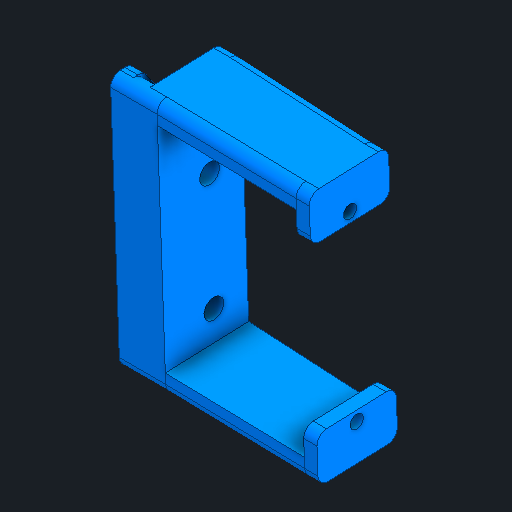
# Autodesk Inventor part: servo_mount
Saved by Autodesk Inventor 2023 (Build 270158030, 158C)
## iProperties
Created: 2022-03-29
Part Number: servo_mount
Material: Generic
Document SubType Name: Modeling
Designer: kardo
Density: 1 g/cm^3
Appearance: Blue Plastic
Author: kardo
Autodesk Inventor part; units mm, degrees
ref_plane "YZ Plane" through (0, 0, 0) normal (1, 0, 0) x (0, 1, 0)
ref_plane "XZ Plane" through (0, 0, 0) normal (0, 1, 0) x (-1, 0, 0)
ref_plane "XY Plane" through (0, 0, 0) normal (0, 0, 1) x (1, 0, 0)
derived "stencil_frame.ipt"
sketch "sk_servo_mount" plane through (-54.6, 0, 0) normal (1, 0, 0) x (0, 1, 0)
  line L0 (-241.5001, 19.2432) -> (11.22, 28.376) construction
  line L1 (-345, 3089.1136) -> (-345, -1866.0023) construction
  line L2 (0, 3089.1136) -> (0, -1866.0023) construction
  line L3 (-195.0558, 20.9216) -> (-195.2941, 27.5173) construction
  line L4 (-195.2941, 27.5173) -> (-177.3059, 28.1674) construction
  line L5 (-177.3059, 28.1674) -> (-177.0675, 21.5717) construction
  point P0 (0, 0)
  point P1 (-186.3, 27.8423)
ref_plane "plane_cowl_left" through (-54.6, 0, 0) normal (1, 0, 0) x (0, 1, 0)
derived "parameters_frame.ipt"
derived "parameters_powertrain.ipt"
derived "parameters_hardware.ipt"
ref_plane "plane_inner_stringer" through (-54.6, -241.5001, 19.2432) normal (1, 0, 0) x (0, 0.9993477, 0.0361144)
ref_plane "plane_fastening" through (-28.6, -241.5001, 19.2432) normal (1, 0, 0) x (0, 0.9993477, 0.0361144)
ref_plane "plane_servo_rod_joint" through (-14.6, -241.5001, 19.2432) normal (1, 0, 0) x (0, 0.9993477, 0.0361144)
sketch "sk_fastening" plane through (-28.6, -241.5001, 19.2432) normal (1, 0, 0) x (0, 0.9993477, 0.0361144)
  line L0 (46.4746, 6.6) -> (64.4746, 6.6) construction
  line L1 (55.4746, 6.6) -> (55.4746, 106.6) construction
  line L2 (55.4746, 106.6) -> (155.4746, 106.6) construction
  line L3 (155.4746, 106.6) -> (155.4746, 22.6) construction
  line L4 (155.4746, 22.6) -> (63.4746, 22.6) construction
  line L5 (63.4746, 22.6) -> (63.4746, 8.6) construction
  line L6 (63.4746, 8.6) -> (58.4746, 8.6) construction
  line L7 (41.9746, 14.6) -> (41.9746, 2.6)
  line L8 (41.9746, 2.6) -> (45.9746, 2.6)
  line L9 (45.9746, 2.6) -> (45.9746, 14.6)
  line L10 (45.9746, 14.6) -> (41.9746, 14.6)
  line L11 (70.9746, 14.6) -> (70.9746, 2.6)
  line L12 (70.9746, 2.6) -> (74.9746, 2.6)
  line L13 (74.9746, 2.6) -> (74.9746, 14.6)
  line L14 (74.9746, 14.6) -> (70.9746, 14.6)
  line L15 (45.9746, 14.6) -> (70.9746, 14.6) construction
  line L16 (70.9746, 2.6) -> (45.9746, 2.6) construction
  line L17 (58.4746, 2.6) -> (58.4746, 14.6) construction
  line L18 (41.9746, 14.6) -> (38.9746, 14.6)
  line L19 (38.9746, 14.6) -> (38.9746, 2.6)
  line L20 (38.9746, 2.6) -> (41.9746, 2.6)
  line L21 (74.9746, 14.6) -> (77.9746, 14.6)
  line L22 (77.9746, 14.6) -> (77.9746, 2.6)
  line L23 (77.9746, 2.6) -> (74.9746, 2.6)
  line L24 (44.4746, 8.6) -> (45.9746, 8.6) construction
  line L25 (70.9746, 8.6) -> (72.4746, 8.6) construction
  point P0 (240.6476, -27.9523)
  dimension "d46" = 100
  dimension "d47" = 84
  dimension "d49" = 100
  dimension "d50" = 92
  dimension "d52" = 14
  dimension "d53" = 5
  dimension "d54" = 25
  dimension "d55" = 33
  dimension "d56" = 3
  dimension "d57" = 3
  dimension "d58" = 12
  dimension "d59" = 28
  constraints: 50 end point, 8 collinear, 8 perpendicular, 7 parallel, 5 midpoint, 2 point on line, 1 coincident, 1 other
  measures "d46" distance of L1.end L2.end
  measures "d47" distance of L2.end L3.end
  measures "d49" distance of L1.start L1.end
  measures "d50" distance of L3.end L4.end
  measures "d52" distance of L4.end L5.end
  measures "d53" distance of L6.end L5.end
  measures "d54" distance between parallel lines of L11 L9
  measures "d55" distance between parallel lines of L13 L7
  measures "d56" distance of L7.start L18.end
  measures "d57" distance of L13.end L21.end
  measures "d58" distance of L21.end L22.end
  measures "d59" distance of L25.end L24.start
sketch "sk_base" plane through (-54.6, -241.5001, 19.2432) normal (1, 0, 0) x (0, 0.9993477, 0.0361144)
  line L0 (41.9746, 14.6) -> (38.9746, 14.6) construction
  line L1 (38.9746, 14.6) -> (38.9746, 2.6) construction
  line L2 (38.9746, 2.6) -> (41.9746, 2.6) construction
  line L3 (77.9746, 2.6) -> (74.9746, 2.6) construction
  line L4 (77.9746, 14.6) -> (77.9746, 2.6) construction
  line L5 (74.9746, 14.6) -> (77.9746, 14.6) construction
  line L6 (46.4746, 6.6) -> (64.4746, 6.6) construction
  line L7 (0, 0) -> (252.8851, 0) construction
  line L8 (38.9746, 1.5) -> (77.9746, 1.5)
  line L9 (77.9746, 1.5) -> (77.9746, 14.1)
  line L10 (77.9746, 14.1) -> (38.9746, 14.1)
  line L11 (38.9746, 14.1) -> (38.9746, 1.5)
  line L12 (46.4746, 6.6) -> (38.9746, 6.6) construction
  line L13 (46.4746, 6.6) -> (46.4746, 14.1) construction
  line L14 (64.4746, 6.6) -> (77.9746, 6.6) construction
  line L15 (64.4746, 6.6) -> (64.4746, 14.1) construction
  point P0 (240.6476, -27.9523)
  point P1 (58.4746, 8.6)
  point P2 (55.4746, 6.6)
  dimension "d60" = 22.5
  dimension "d61" = 16.5
  dimension "d62" = 18
  dimension "d64" = 1.5
  dimension "d65" = 7.5
  dimension "d66" = 16.5
  dimension "d67" = 22.5
  constraints: 16 end point, 6 perpendicular, 4 point on line, 2 parallel
  measures "d60" distance from line of L4 point (55.475, 6.6)
  measures "d61" distance from line of L1 point (55.475, 6.6)
  measures "d62" distance of L6.start L6.end
  measures "d64" distance between parallel lines of L7 L8
  measures "d65" distance of L12.start L13.end
  measures "d66" distance from line of point (55.475, 6.6) L11
  measures "d67" distance from line of point (55.475, 6.6) L9
ref_plane "plane_column_bottom" through (-52.1, -241.5001, 19.2432) normal (1, 0, 0) x (0, 0.9993477, 0.0361144)
ref_plane "plane_outer_plate" through (-57.1, -241.5001, 19.2432) normal (1, 0, 0) x (0, 0.9993477, 0.0361144)
sketch "sk_hex_holes" plane through (-57.1, -241.5001, 19.2432) normal (1, 0, 0) x (0, 0.9993477, 0.0361144)
  line L0 (48.0624, 9.35) -> (49.6501, 6.6)
  line L1 (49.6501, 6.6) -> (48.0624, 3.85)
  line L2 (48.0624, 3.85) -> (44.8869, 3.85)
  line L3 (44.8869, 3.85) -> (43.2992, 6.6)
  line L4 (43.2992, 6.6) -> (44.8869, 9.35)
  line L5 (44.8869, 9.35) -> (48.0624, 9.35)
  line L6 (66.0624, 9.35) -> (67.6501, 6.6)
  line L7 (67.6501, 6.6) -> (66.0624, 3.85)
  line L8 (66.0624, 3.85) -> (62.8869, 3.85)
  line L9 (62.8869, 3.85) -> (61.2992, 6.6)
  line L10 (61.2992, 6.6) -> (62.8869, 9.35)
  line L11 (62.8869, 9.35) -> (66.0624, 9.35)
  point P0 (240.6476, -27.9523)
  point P1 (46.4746, 6.6)
  point P2 (64.4746, 6.6)
  point P3 (46.4746, 6.6)
  point P4 (64.4746, 6.6)
  dimension "d102" = 5.5
  constraints: 24 end point, 2 coincident, 2 collinear, 26 other
  measures "d102" distance between parallel lines of L2 L5
sketch "sk_bridge" plane through (-54.6, -241.5001, 19.2432) normal (1, 0, 0) x (0, 0.9993477, 0.0361144)
  line L0 (77.9746, 14.1) -> (38.9746, 14.1) projected
  line L1 (38.9746, 14.1) -> (38.9746, 1.5) projected
  line L2 (77.9746, 1.5) -> (77.9746, 14.1) projected
  line L3 (38.9746, 11.1) -> (77.9746, 11.1)
  point P0 (240.6476, -27.9523)
  dimension "d70" = 3
  constraints: 2 end point, 2 point on line, 1 parallel
  measures "d70" distance between parallel lines of L0 L3
sketch "sk_backplate" plane through (-57.1, -241.5001, 19.2432) normal (1, 0, 0) x (0, 0.9993477, 0.0361144)
  line L0 (38.9746, 14.1) -> (38.9746, 1.5) construction
  line L1 (77.9746, 14.1) -> (38.9746, 14.1) projected
  line L2 (77.9746, 1.5) -> (77.9746, 14.1) construction
  line L3 (66.0624, 3.85) -> (62.8869, 3.85) projected
  line L4 (48.0624, 3.85) -> (44.8869, 3.85) projected
  line L5 (77.9746, 14.1) -> (77.9746, 11.1)
  line L6 (69.2378, 3.85) -> (66.0624, 3.85)
  line L7 (62.8869, 3.85) -> (48.0624, 3.85)
  line L8 (44.8869, 3.85) -> (41.7115, 3.85)
  line L9 (38.9746, 14.1) -> (38.9746, 11.1)
  line L10 (44.8869, 3.85) -> (43.2992, 6.6) construction
  line L11 (38.9746, 11.1) -> (77.9746, 11.1) construction
  line L12 (67.6501, 6.6) -> (66.0624, 3.85) construction
  line L13 (41.7115, 3.85) -> (40.1238, 6.6)
  line L14 (40.1238, 6.6) -> (38.9746, 11.1)
  line L15 (77.9746, 11.1) -> (70.8255, 6.6)
  line L16 (70.8255, 6.6) -> (69.2378, 3.85)
  point P0 (240.6476, -27.9523)
  constraints: 18 end point, 4 equal length, 2 collinear, 2 parallel
ref_plane "plane_column_top" through (-30.6, -241.5001, 19.2432) normal (1, 0, 0) x (0, 0.9993477, 0.0361144)
extrude "extrude_fastening_plates" add sketch "sk_fastening" against normal up to surface (2 mm away)
extrude "extrude_backplate" add sketch "sk_backplate" against normal blind 2
extrude "extrude_front_plate" add sketch "sk_base" along normal up to surface (2.5 mm away)
extrude "extrude_bridge" add sketch "sk_bridge" against normal up to surface (2.5 mm away)
sketch "sk_column_bottom_1" plane through (-52.1, -241.5001, 19.2432) normal (1, 0, 0) x (0, 0.9993477, 0.0361144)
  line L0 (77.9746, 14.1) -> (38.9746, 14.1) construction
  line L1 (38.9746, 1.5) -> (77.9746, 1.5) construction
  line L2 (41.9746, 14.6) -> (41.9746, 2.6) construction
  line L3 (38.9746, 14.6) -> (38.9746, 2.6) construction
  line L4 (38.9746, 14.1) -> (41.9746, 14.1)
  line L5 (41.9746, 14.1) -> (41.9746, 1.5)
  line L6 (41.9746, 1.5) -> (38.9746, 1.5)
  line L7 (38.9746, 1.5) -> (38.9746, 14.1)
  point P0 (240.6476, -27.9523)
  constraints: 8 end point, 4 collinear
sketch "sk_column_top_1" plane through (-30.6, -241.5001, 19.2432) normal (1, 0, 0) x (0, 0.9993477, 0.0361144)
  line L0 (38.9746, 14.6) -> (38.9746, 2.6) projected
  line L1 (41.9746, 14.6) -> (38.9746, 14.6) projected
  line L2 (41.9746, 14.6) -> (41.9746, 2.6) projected
  line L3 (38.9746, 2.6) -> (41.9746, 2.6) projected
  point P0 (240.6476, -27.9523)
sketch "sk_column_bottom_2" plane through (-52.1, -241.5001, 19.2432) normal (1, 0, 0) x (0, 0.9993477, 0.0361144)
  line L0 (74.9746, 2.6) -> (74.9746, 14.6) construction
  line L1 (77.9746, 14.6) -> (77.9746, 2.6) construction
  line L2 (77.9746, 14.1) -> (38.9746, 14.1) construction
  line L3 (38.9746, 1.5) -> (77.9746, 1.5) construction
  line L4 (74.9746, 14.1) -> (74.9746, 1.5)
  line L5 (74.9746, 1.5) -> (77.9746, 1.5)
  line L6 (77.9746, 1.5) -> (77.9746, 14.1)
  line L7 (77.9746, 14.1) -> (74.9746, 14.1)
  point P0 (240.6476, -27.9523)
  constraints: 8 end point, 4 collinear
sketch "sk_column_top_2" plane through (-30.6, -241.5001, 19.2432) normal (1, 0, 0) x (0, 0.9993477, 0.0361144)
  line L0 (74.9746, 2.6) -> (74.9746, 14.6) projected
  line L1 (77.9746, 14.6) -> (77.9746, 2.6) projected
  line L2 (74.9746, 14.6) -> (77.9746, 14.6) projected
  line L3 (77.9746, 2.6) -> (74.9746, 2.6) projected
  point P0 (240.6476, -27.9523)
loft "column_1" add profiles "sk_column_bottom_1", "sk_column_top_1"
loft "column_2" add profiles "sk_column_bottom_2", "sk_column_top_2"
hole "fastening_holes" at (-28.6, -197.3651, 29.4438) at (-28.6, -169.3833, 30.455) direction (-1, 0, 0) diameter 2 depth 2 tip angle 118
hole "stringer_holes" at (-54.6, -177.3059, 28.1674) at (-54.6, -195.2941, 27.5173) direction (1, 0, 0) diameter 3 depth 2.5 tip angle 118
extrude "hex_holes" cut sketch "sk_hex_holes" against normal through all
fillet "fillet_outer_corners" radius 1.5 16 edges at (-41.35, -203.0691, 34.9914) (-41.35, -202.6249, 22.6994) (-29.6, -202.6448, 23.2491) (-53.35, -202.6051, 22.1498) (-29.6, -203.0782, 35.2412) (-29.6, -164.1036, 36.6497) (-41.35, -164.0946, 36.3999) (-55.6, -164.0855, 36.15) (-29.6, -163.6702, 24.6575) (-41.35, -163.6504, 24.1079) (-53.35, -163.6305, 23.5582) (-29.6, -196.0827, 35.494) (-29.6, -195.6493, 23.5019) (-29.6, -171.099, 36.3969) (-29.6, -170.6657, 24.4047) (-55.6, -203.0601, 34.7416)
fillet "fillet_backplate" radius 1.5 8 edges at (-58.1, -163.9772, 33.152) (-55.85, -163.9772, 33.152) (-58.1, -170.9592, 28.3967) (-58.1, -172.4465, 25.5912) (-58.1, -199.9548, 24.5971) (-58.1, -201.6408, 27.2879) (-58.1, -202.9518, 31.7435) (-55.85, -202.9518, 31.7435)
equation "\"d52\" = servo_arm_length"
equation "\"d53\" = servo_axis_location"
equation "\"d55\" = servo_length_fastening"
equation "\"d58\" = servo_width"
equation "\"d59\" = servo_fastening_distance"
equation "\"d88\" = servo_fastening_diam"
equation "\"d95\" = drill_servo_mount_diam"
equation "\"d44\" = servo_height_fastening - servo_height_joint"
equation "\"servo_arm_length\" = 14"
equation "\"servo_axis_location\" = 5"
equation "\"servo_length_fastening\" = 33"
equation "\"servo_width\" = 12"
equation "\"servo_fastening_distance\" = 28"
equation "\"servo_fastening_diam\" = 2"
equation "\"drill_servo_mount_diam\" = 3"
equation "\"servo_height_fastening\" = 20"
equation "\"servo_height_joint\" = 34"
body "Solid2"
